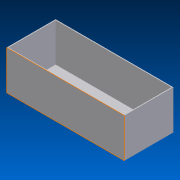
# Autodesk Inventor part: super large Battery Box Pastic 4
Saved by Autodesk Inventor 2012 (Build 160160000, 160)
## iProperties
Created: 2012-07-01
Part Number: super large Battery Box Pastic 4
Material: Default
Document SubType Name: Modeling
Designer: Hemant
Density: 1 g/cm^3
Author: Hemant
Autodesk Inventor part; units mm, degrees
ref_plane "YZ Plane" through (0, 0, 0) normal (1, 0, 0) x (0, 1, 0)
ref_plane "XZ Plane" through (0, 0, 0) normal (0, 1, 0) x (-1, 0, 0)
ref_plane "XY Plane" through (0, 0, 0) normal (0, 0, 1) x (1, 0, 0)
sketch "Sketch1" plane through (0, 0, 0) normal (0, 0, 1) x (1, 0, 0)
  line L0 (0, 0) -> (847.725, 0)
  line L1 (847.725, 0) -> (847.725, 282.575)
  line L2 (847.725, 282.575) -> (0, 282.575)
  line L3 (0, 282.575) -> (0, 0)
  dimension "d0" = 847.725
  dimension "d1" = 282.575
  constraints: 8 end point, 2 parallel, 1 horizontal, 1 perpendicular
  measures "d0" distance between parallel lines of L1 L3
  measures "d1" distance between parallel lines of L2 L0
extrude "Extrusion1" add sketch "Sketch1" along normal blind 352.425
sketch "Sketch2" plane through (0, 282.575, 0) normal (0, 1, 0) x (1, 0, 0)
  line L0 (0, -352.425) -> (847.725, -352.425) projected
  line L1 (0, 0) -> (0, -352.425) projected
  line L2 (6.35, -346.075) -> (841.375, -346.075)
  line L3 (841.375, -346.075) -> (841.375, -6.35)
  line L4 (841.375, -6.35) -> (6.35, -6.35)
  line L5 (6.35, -6.35) -> (6.35, -346.075)
  dimension "d4" = 6.35
  dimension "d5" = 6.35
  dimension "d6" = 835.025
  dimension "d7" = 339.725
  constraints: 8 end point, 2 parallel, 1 horizontal, 1 perpendicular
  measures "d4" distance between parallel lines of L5 L1
  measures "d5" distance between parallel lines of L0 L2
  measures "d6" distance between parallel lines of L3 L5
  measures "d7" distance between parallel lines of L4 L2
extrude "Extrusion2" cut sketch "Sketch2" against normal blind 276.225
sketch "Sketch3" plane through (0, 0, 352.425) normal (0, 0, 1) x (1, 0, 0)
  line L0 (0, 0) -> (0, 282.575) projected
  line L1 (847.725, 0) -> (0, 0) projected
  line L2 (847.725, 282.575) -> (847.725, 0) projected
  line L3 (0, 282.575) -> (847.725, 282.575) projected
body "Solid1"
